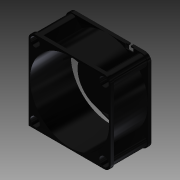
# Autodesk Inventor part: fan body
Saved by Autodesk Inventor 2014 SP1 (Build 180222100, 222)
## iProperties
Category: Electrical
Company: Autodesk Inc.
Shininess: 64.0
Length Units: 11272
Angle Units: 11279
Time Units: 11290
Mass Units: 11286
Length Display Precision: 3
Angle Display Precision: 2
Compacted: True
Part Number: fan body
Document SubType Name: Modeling
Created: 2012-11-26
Designer: Autodesk Inc.
Density: 1 g/cm^3
Material: Generic
Mass: 5.49502 g
Surface Area: 95.2958 cm^2
Volume: 5.49502 cm^3
Appearance: Glossy - Black
Density: 0.0
Volumn: 0.0
Area: 0.0
PropertySet Name: Model Information
Control State: 0
Master: False
Checked Out: False
Author: Autodesk Inc.
Autodesk Inventor part; units mm, degrees
ref_plane "YZ Plane" through (0, 0, 0) normal (1, 0, 0) x (0, 1, 0)
sketch "Sketch1" plane through (0, 0, 0) normal (0, 0, 1) x (1, 0, 0)
  line L0 (0, 0) -> (39.878, 0)
  line L1 (39.878, 0) -> (39.878, 39.878)
  line L2 (39.878, 39.878) -> (0, 39.878)
  line L3 (0, 39.878) -> (0, 0)
  dimension "d0" = 39.878
  dimension "d1" = 39.878
  constraints: 8 end point, 2 parallel, 1 horizontal, 1 perpendicular
  measures "d0" distance of L0.end L1.end
  measures "d1" distance of L1.end L2.end
extrude "Extrusion1" add sketch "Sketch1" along normal blind 19.812
ref_plane "Work Plane1" through (19.939, 0, 0) normal (1, 0, 0) x (0, 0, -1)
sketch "Sketch2" plane through (19.939, 0, 0) normal (1, 0, 0) x (0, 0, -1)
  line L0 (-19.812, 39.878) -> (-19.812, 0) projected
  line L1 (0, 0) -> (0, 39.878) projected
  line L2 (-19.812, 19.939) -> (0, 19.939)
  line L3 (-18.1102, 52.578) -> (-1.7018, 52.578)
  line L4 (-1.7018, 52.578) -> (-1.7018, 39.878)
  line L5 (-1.7018, 39.878) -> (-18.1102, 39.878)
  line L6 (-18.1102, 39.878) -> (-18.1102, 52.578)
  line L7 (-19.812, 39.878) -> (0, 39.878)
  dimension "d4" = 1.7018
  dimension "d5" = 1.7018
  dimension "d6" = 12.7
  constraints: 12 end point, 2 midpoint, 2 parallel, 2 perpendicular, 1 collinear, 1 horizontal
  measures "d4" distance between parallel lines of L0 L6
  measures "d5" distance between parallel lines of L1 L4
  measures "d6" distance between parallel lines of L3 L5
revolve "Revolution1" cut sketch "Sketch2" angle 360 about axis through (19.939, 19.939, 19.812) along (0, 0, -1) contours L6 L3 L4 L5
fillet "Fillet1" radius 3.175 7 edges at (39.878, 39.878, 18.9611) (39.878, 39.878, 0.8509) (0, 39.878, 18.9611) (0, 39.878, 0.8509) (0, 0, 0.8509) (39.878, 0, 0.8509) (39.878, 0, 18.9611)
sketch "Sketch3" plane through (0, 0, 19.812) normal (0, 0, 1) x (1, 0, 0)
  arc A0 (39.878, 36.703) -> (36.703, 39.878) centre (36.703, 36.703) ccw projected
  circle A1 centre (36.703, 36.703) radius 2.286
  dimension "d9" = 4.572
  constraints: 1 centre point, 1 coincident, 1 concentric
  measures "d9" diameter of A1
extrude "Extrusion2" cut sketch "Sketch3" against normal through all
sketch "Sketch4" plane through (19.939, 39.878, 1.7018) normal (0, 0, 1) x (1, 0, 0)
  circle A0 centre (16.764, -3.175) radius 2.286 projected
  arc A1 (19.939, -3.175) -> (16.764, 0) centre (16.764, -3.175) ccw projected
  arc A2 (19.939, -19.939) -> (0, 0) centre (0, -19.939) ccw projected
  line L0 (16.764, -3.175) -> (0, -19.939)
  circle A3 centre (16.764, -3.175) radius 2.7094
  line L1 (18.6798, -5.0908) -> (15.8841, -7.8866)
  line L2 (14.8482, -1.2592) -> (12.0524, -4.0549)
  constraints: 6 end point, 4 point on circle, 2 parallel, 2 tangent, 1 centre point, 1 coincident, 1 concentric
extrude "Extrusion3" add sketch "Sketch4" along normal up to next
pattern_circular "Circular Pattern1" count 4 over 360 about axis through (19.939, 19.939, 9.906) along (0, 0, 1) of "Extrusion2", "Extrusion3"
sketch "Sketch5" plane through (0, 0, 19.812) normal (0, 0, 1) x (1, 0, 0)
  arc A0 (19.939, 39.878) -> (7.8866, 35.8231) centre (19.939, 19.939) ccw projected
  arc A1 (31.9914, 35.8231) -> (19.939, 39.878) centre (19.939, 19.939) ccw projected
  arc A2 (31.9914, 35.8231) -> (19.939, 39.878) centre (19.939, 19.939) ccw projected
  arc A3 (19.939, 39.878) -> (7.8866, 35.8231) centre (19.939, 19.939) ccw projected
  circle A4 centre (19.939, 19.939) radius 19.2405
  dimension "d19" = 38.481
  constraints: 1 centre point, 1 coincident, 1 concentric
  measures "d19" diameter of A4
extrude "Extrusion4" cut sketch "Sketch5" against normal through all
sketch "Sketch6" plane through (0, 0, 0) normal (0, 0, -1) x (-1, 0, 0)
  circle A0 centre (-19.939, 19.939) radius 19.2405 projected
  circle A1 centre (-36.703, 3.175) radius 2.286 projected
  line L0 (-15.6996, 8.562) -> (-35.9048, 1.0329)
  line L1 (-19.5524, 7.804) -> (-34.6449, 2.18)
  line L2 (-12.546, 29.5698) -> (-0.7061, 20.4811)
  line L3 (-9.8588, 26.7065) -> (-0.7003, 19.6761)
  arc A2 (-12.546, 29.5698) -> (-19.5524, 7.804) centre (-19.939, 19.939) ccw
  arc A3 (-15.6996, 8.562) -> (-9.8588, 26.7065) centre (-19.939, 19.939) ccw
  dimension "d21" = 0.635
  dimension "d23" = 0.635
  constraints: 8 end point, 8 point on circle, 3 tangent, 2 centre point, 1 coincident
  measures "d21" distance between parallel lines of L1 L0
  measures "d23" distance between parallel lines of L3 L2
extrude "fan support1" add sketch "Sketch6" against normal blind 3.81 contours A0 L3 A3 L0 L1 A2 L2 | A0 L0 A1 L1
sketch "Sketch7" plane through (0, 0, 0) normal (0, 0, -1) x (-1, 0, 0)
  arc A0 (-12.546, 29.5698) -> (-19.5524, 7.804) centre (-19.939, 19.939) ccw projected
  arc A1 (-0.7061, 20.4811) -> (-30.3715, 3.7724) centre (-19.939, 19.939) ccw projected
  line L0 (-36.703, 39.878) -> (-3.175, 39.878) projected
  line L1 (-39.878, 3.175) -> (-39.878, 36.703) projected
  line L2 (-33.4114, 39.878) -> (-33.4114, 23.4993)
  line L3 (-28.3314, 39.878) -> (-28.3314, 29.7703)
  line L4 (-19.939, 19.939) -> (-32.8458, 27.844)
  line L5 (-33.4114, 23.4993) -> (-31.8038, 22.5147)
  line L6 (-28.3314, 29.7703) -> (-27.625, 29.3377)
  dimension "d26" = 5.08
  dimension "d27" = 8.001
  dimension "d28" = 4.0005
  constraints: 10 end point, 4 parallel, 2 point on circle, 2 point on line
  measures "d26" distance between parallel lines of L2 L3
  measures "d27" distance between parallel lines of L6 L5
  measures "d28" distance between parallel lines of L4 L6
extrude "fan support2" add sketch "Sketch7" against normal blind 1.5875
sketch "Sketch8" plane through (0, 0, 0) normal (0, 0, -1) x (-1, 0, 0)
  line L0 (-33.4114, 33.6755) -> (-33.4114, 23.4993) projected
  line L1 (-33.4114, 23.4993) -> (-31.8038, 22.5147) projected
  line L2 (-28.3314, 29.7703) -> (-28.3314, 37.2527) projected
  line L3 (-36.703, 39.878) -> (-3.175, 39.878) projected
  line L4 (0, 36.703) -> (0, 3.175) projected
  arc A0 (-15.6996, 8.562) -> (-9.8588, 26.7065) centre (-19.939, 19.939) ccw projected
  line L5 (-31.0281, 22.7842) -> (-32.7764, 23.855)
  line L6 (-32.7764, 23.855) -> (-32.7764, 39.243)
  line L7 (-32.7764, 39.243) -> (-28.9664, 39.243)
  circle A1 centre (-19.939, 19.939) radius 11.4483
  line L8 (-28.9664, 39.243) -> (-28.9664, 26.9796)
  dimension "d31" = 22.8966
  dimension "d32" = 0.635
  dimension "d33" = 0.635
  dimension "d34" = 0.635
  dimension "d35" = 0.635
  constraints: 8 end point, 2 parallel, 2 perpendicular, 2 point on circle, 1 centre point, 1 coincident, 1 concentric
  measures "d31" diameter of A1
  measures "d32" distance from line of L1 L5.end
  measures "d33" distance between parallel lines of L0 L6
  measures "d34" distance between parallel lines of L2 L8
  measures "d35" distance between parallel lines of L3 L7
extrude "fan support3" cut sketch "Sketch8" against normal blind 1.27 contours L5 L6 L7 L8 A1
sketch "Sketch9" plane through (0, 0, 1.27) normal (0, 0, -1) x (-1, 0, 0)
  line L0 (-32.7764, 39.243) -> (-32.7764, 23.855) projected
  line L1 (-32.7764, 37.9276) -> (-28.9664, 37.9276)
  line L2 (-28.9664, 37.9276) -> (-28.9664, 40.5886)
  line L3 (-28.9664, 40.5886) -> (-32.7764, 40.5886)
  line L4 (-32.7764, 40.5886) -> (-32.7764, 37.9276)
  constraints: 8 end point, 2 parallel, 1 horizontal, 1 perpendicular, 1 point on line
extrude "fan support4" cut sketch "Sketch9" against normal blind 1.5557
sketch "Sketch10" plane through (0, 0, 0) normal (0, 0, -1) x (-1, 0, 0)
  line L0 (-32.7764, 39.243) -> (-28.9664, 39.243) projected
  line L1 (-36.703, 39.878) -> (-3.175, 39.878) projected
  line L2 (-31.1757, 39.878) -> (-29.8511, 39.878)
  line L3 (-29.8511, 39.878) -> (-29.8511, 39.243)
  line L4 (-29.8511, 39.243) -> (-31.1757, 39.243)
  line L5 (-31.1757, 39.243) -> (-31.1757, 39.878)
  constraints: 8 end point, 2 parallel, 2 point on line, 1 horizontal, 1 perpendicular
extrude "fan support5" cut sketch "Sketch10" against normal blind 1.5557
ref_plane "fan interface" through (0, 0, 5.3975) normal (0, 0, 1) x (1, 0, 0)
equation "\"d5\" = d4"
equation "\"d28\" = 0.5 * d27"
equation "\"d33\" = d32"
equation "\"d34\" = d33"
equation "\"d35\" = d34"
body "Solid1"
